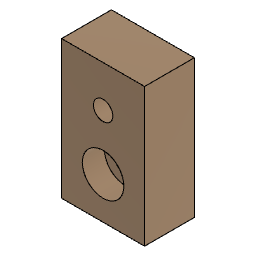
Standoff TR (Autodesk Fusion 360 design; units mm, degrees)
Autodesk Fusion 360 part; units mm, degrees
sketch "Front" plane through (0, 0, 0) normal (0, 1, 0) x (1, 0, 0)
  line L0 (-15, -25) -> (15, -25)
  line L1 (15, -25) -> (15, 25)
  line L2 (15, 25) -> (-15, 25)
  line L3 (-15, 25) -> (-15, -25)
  line L4 (0, -25) -> (0, 25) construction
  circle A0 centre (0, 10) radius 4
  circle A1 centre (0, -10) radius 3.5
  circle A2 centre (0, 10) radius 7.5
  dimension "d11" = 30
  dimension "d12" = 50
  dimension "d19" = 8
  dimension "d20" = 7
  dimension "d21" = 20
  dimension "d24" = 15
  dimension "d26" = 15
  constraint horizontal L0
  constraint vertical L1
  constraint horizontal L2
  constraint vertical L3
  constraint midpoint L0 L4.start
  constraint midpoint L2 L4.end
  constraint coincident L4 A0.centre
  constraint coincident L4 A1.centre
  constraint concentric A0 A2
  measures "d11" distance of L0.start L0.end
  measures "d12" distance of L0.start L2.end
  measures "d19" diameter of A0
  measures "d20" diameter of A1
  measures "d21" distance of A0.centre A1.centre
  measures "d24" distance of L2 A0.centre
  measures "d26" diameter of A2
extrude "Extrude3" add sketch "Front" against normal blind 10 contours A2
extrude "Extrude4" add sketch "Front" against normal blind 18 contours L0 L1 L2 L3
named bodies: "Standoff TR"
